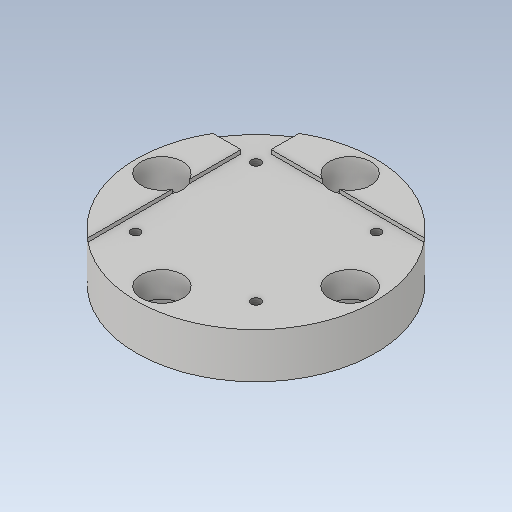
# Autodesk Inventor part: FAB-OX0005
Saved by Autodesk Inventor 2020 (Build 240168000, 168)
## iProperties
Created: 2017-01-09
Part Number: FAB-OX0005
Material: Generic
Document SubType Name: Modeling
Designer: map
Density: 1 g/cm^3
Appearance: Default
Description: Goniometer spacer
Author: map
Revision Number: 02
Autodesk Inventor part; units mm, degrees
ref_plane "YZ Plane" through (0, 0, 0) normal (1, 0, 0) x (0, 1, 0)
ref_plane "XZ Plane" through (0, 0, 0) normal (0, 1, 0) x (-1, 0, 0)
ref_plane "XY Plane" through (0, 0, 0) normal (0, 0, 1) x (1, 0, 0)
sketch "Sketch1" plane through (0, 0, 0) normal (0, 1, 0) x (-1, 0, 0)
  circle A0 centre (0, 0) radius 25 construction
  line L0 (44.45, 0) -> (-44.45, 0) construction
  line L1 (0, -44.45) -> (0, 44.45) construction
  circle A1 centre (0, 0) radius 31.75
  circle A2 centre (0, 0) radius 16 construction
  line L2 (11.3137, 11.3137) -> (-11.3137, -11.3137) construction
  line L3 (-11.3137, 11.3137) -> (11.3137, -11.3137) construction
  line L4 (-20, 20) -> (20, 20) construction
  line L5 (20, 20) -> (20, -20) construction
  line L6 (20, -20) -> (-20, -20) construction
  line L7 (-20, -20) -> (-20, 20) construction
  line L8 (-20, 20) -> (20, -20) construction
  line L9 (20, 20) -> (-20, -20) construction
  line L10 (16, -20) -> (16, -27.4238)
  line L11 (16, -20) -> (-24.6589, -20)
  line L12 (20, -16) -> (27.4238, -16)
  line L13 (20, -16) -> (20, 24.6589)
  line L14 (16, -16) -> (-16, -16)
  line L15 (-16, -16) -> (-16, 16)
  line L16 (-16, 16) -> (16, 16)
  line L17 (16, 16) -> (16, -16)
  point P0 (0, 25)
  point P1 (25, 0)
  point P2 (0, -25)
  point P3 (-25, 0)
  point P4 (-16, 16)
  dimension "M6ClearancePatternDiameter" = 50
  dimension "diameter" = 63.5
  dimension "M3TappedPatternEdge" = 32
  dimension "d3" = 45
  dimension "d20" = 40
  dimension "d21" = 40
  constraints: 32 end point, 12 point on circle, 8 point on line, 7 coincident, 6 perpendicular, 4 parallel, 4 tangent, 3 centre point, 2 horizontal, 2 line through centre, 2 midpoint, 1 collinear
  measures "M6ClearancePatternDiameter" diameter of A0
  measures "diameter" diameter of A1
  measures "M3TappedPatternEdge" diameter of A2
  measures "d3" angle of L2 L1
  measures "d20" distance of L5.end L6.end
  measures "d21" distance of L4.end L5.end
extrude "Extrusion1" add sketch "Sketch1" against normal blind 12 contours A1 L12 L13 | L13 L12 A1 L10 L11 | L11 L10 A1 | L14 L15 L16 L17
extrude "Extrusion3" add sketch "Sketch1" along normal blind 1 contours A1 L12 L13 | L11 L10 A1
hole "M3Tapped" at (-16, 0, -16) at (16, 0, -16) at (16, 0, 16) at (-16, 0, 16) direction (0, -1, 0) diameter 2.459 depth 8.8 tip angle 118 thread size "M3x0.5" class "6H" standard "ISO Metric profile"
hole "Hole4" at (0, 0, 25) at (-25, 0, 0) at (0, 0, -25) at (25, 0, 0) direction (0, -1, 0) diameter 6.4 end through all counterbore diameter 11 counterbore depth 6.8 clearance for "Socket Head Cap Screw ISO 4762" size "M6" standard "ISO"
sketch "Sketch2" plane through (0, 0, 0) normal (0, -1, 0) x (1, 0, 0)
  circle A0 centre (25, 0) radius 5.5 projected
  arc A1 (2.2913, -20) -> (-2.2913, -20) centre (0, -25) ccw projected
  arc A2 (-2.2913, -20) -> (2.2913, -20) centre (0, -25) ccw projected
  circle A3 centre (0, 25) radius 5.5 projected
  line L0 (-20, 24.6589) -> (-20, 2.2913) projected
  line L1 (-20, 2.2913) -> (-20, -2.2913) projected
  line L2 (-20, -2.2913) -> (-20, -16) projected
  line L3 (-20, -16) -> (-27.4238, -16) projected
  line L4 (-16, -27.4238) -> (-16, -20) projected
  line L5 (-16, -20) -> (-2.2913, -20) projected
  line L6 (-2.2913, -20) -> (2.2913, -20) projected
  line L7 (2.2913, -20) -> (24.6589, -20) projected
  arc A4 (-20, -2.2913) -> (-20, 2.2913) centre (-25, 0) ccw projected
  arc A5 (-20, 2.2913) -> (-20, -2.2913) centre (-25, 0) ccw projected
  arc A6 (-27.4238, -16) -> (-16, -27.4238) centre (0, 0) ccw projected
  arc A7 (-16, -27.4238) -> (24.6589, -20) centre (0, 0) ccw projected
  arc A8 (-20, 24.6589) -> (-27.4238, -16) centre (0, 0) ccw projected
  arc A9 (24.6589, -20) -> (-20, 24.6589) centre (0, 0) ccw projected
  circle A10 centre (16, 16) radius 1.2295 projected
  circle A11 centre (-16, -16) radius 1.2295 projected
  circle A12 centre (16, -16) radius 1.2295 projected
  circle A13 centre (-16, 16) radius 1.2295 projected
extrude "Extrusion4" cut sketch "Sketch2" against normal through all contours A2 L6 | L1 A5
equation "\"d21\" = d20"
equation "\"d4\" = thickness"
equation "\"d24\" = recessDepth"
equation "\"d40\" = recessDepth"
equation "\"thickness\" = 12"
equation "\"recessDepth\" = 1"
body "Solid1"
